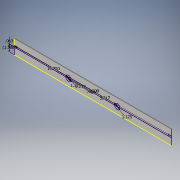
# Autodesk Inventor part: OutsidePlate
Saved by Autodesk Inventor 2016 (Build 200138000, 138)
## iProperties
Created: 2017-01-19
Part Number: OutsidePlate
Material: Generic
Document SubType Name: Modeling
Designer: Kyle
Density: 1 g/cm^3
Appearance: Default
Author: Kyle
Autodesk Inventor part; units mm, degrees
ref_plane "YZ Plane" through (0, 0, 0) normal (1, 0, 0) x (0, 1, 0)
ref_plane "XZ Plane" through (0, 0, 0) normal (0, 1, 0) x (-1, 0, 0)
ref_plane "XY Plane" through (0, 0, 0) normal (0, 0, 1) x (1, 0, 0)
sketch "Sketch1" plane through (0, 0, 0) normal (0, 0, 1) x (1, 0, 0)
  line L0 (0, 0) -> (850.9, 0)
  line L1 (850.9, 0) -> (850.9, 76.2)
  line L2 (850.9, 76.2) -> (0, 76.2)
  line L3 (0, 76.2) -> (0, 0)
  dimension "d0" = 850.9
  dimension "d1" = 76.2
  constraints: 8 end point, 2 parallel, 1 horizontal, 1 perpendicular
  measures "d0" distance of L2.end L1.end
  measures "d1" distance of L1.end L0.end
extrude "Extrusion1" add sketch "Sketch1" along normal blind 3.175
sketch "Sketch2" plane through (0, 0, 3.175) normal (0, 0, 1) x (1, 0, 0)
  line L0 (0, 0) -> (850.9, 0) projected
  line L1 (0, 0) -> (0, 38.1)
  line L2 (0, 76.2) -> (0, 0) projected
  line L3 (0, 38.1) -> (0, 36.5125)
  line L4 (0, 36.5125) -> (850.9, 36.5125)
  line L5 (0, 36.5125) -> (425.45, 36.5125)
  line L6 (425.45, 36.5125) -> (292.9509, 36.5125)
  line L7 (425.45, 36.5125) -> (557.9491, 36.5125)
  circle A0 centre (292.9509, 36.5125) radius 14.2875
  circle A1 centre (557.9491, 36.5125) radius 14.2875
  dimension "d4" = 38.1
  dimension "d5" = 1.5875
  dimension "d6" = 850.9
  dimension "d7" = 425.45
  dimension "d8" = 132.4991
  dimension "d9" = 132.4991
  dimension "d10" = 28.575
  dimension "d11" = 28.575
  constraints: 12 end point, 3 point on line, 2 centre point, 2 coincident, 2 midpoint, 1 horizontal
  measures "d4" distance of L0.start L1.end
  measures "d5" distance of L1.end L3.end
  measures "d6" distance of L3.end L4.end
  measures "d7" distance of L3.end L5.end
  measures "d8" distance of L5.end L6.end
  measures "d9" distance of L5.end L7.end
  measures "d10" diameter of A0
  measures "d11" diameter of A1
body "Solid1"
